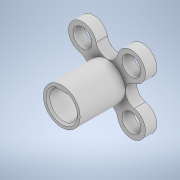
# Autodesk Inventor part: teenee_part
Saved by Autodesk Inventor 2020 (Build 240168000, 168)
## iProperties
Created: 2019-04-24
Part Number: teenee_part
Material: Generic
Document SubType Name: Modeling
Designer: Connor
Density: 1 g/cm^3
Appearance: Default
Author: Connor
Autodesk Inventor part; units mm, degrees
ref_plane "YZ Plane" through (0, 0, 0) normal (1, 0, 0) x (0, 1, 0)
ref_plane "XZ Plane" through (0, 0, 0) normal (0, 1, 0) x (-1, 0, 0)
ref_plane "XY Plane" through (0, 0, 0) normal (0, 0, 1) x (1, 0, 0)
sketch "Sketch1" plane through (0, 0, 0) normal (0, 0, 1) x (1, 0, 0)
  line L0 (-12.5, 12.5) -> (12.5, 12.5)
  line L1 (12.5, 12.5) -> (12.5, -12.5)
  line L2 (12.5, -12.5) -> (-12.5, -12.5)
  line L3 (-12.5, -12.5) -> (-12.5, 12.5)
  line L4 (-12.5, 12.5) -> (12.5, -12.5) construction
  line L5 (-12.5, -12.5) -> (12.5, 12.5) construction
  arc A0 (-1.7861, 2.625) -> (1.7861, 2.625) centre (0, 0) ccw
  line L6 (-1.7861, 2.625) -> (1.7861, 2.625)
  circle A1 centre (-6.5, 6.5) radius 2.5
  circle A2 centre (6.5, 6.5) radius 2.5
  circle A3 centre (6.5, -6.5) radius 2.5
  circle A4 centre (-6.5, -6.5) radius 2.5
  line L7 (1.9339, 3.125) -> (-1.9339, 3.125)
  arc A5 (-1.9339, 3.125) -> (1.9339, 3.125) centre (0, 0) ccw
  point P0 (0, 0)
  dimension "d0" = 6.35
  dimension "d1" = 25
  dimension "d2" = 5.8
  dimension "d3" = 5
  dimension "d6" = 13
  dimension "d7" = 0.5
  constraints: 16 end point, 6 centre point, 4 point on circle, 4 point on line, 3 equal radius, 2 coincident, 2 horizontal, 2 horizontal alignment, 2 parallel, 2 perpendicular, 1 midpoint, 1 vertical alignment, 1 other
  measures "d0" diameter of A0
  measures "d1" distance between parallel lines of L1 L3
  measures "d3" diameter of A1
  measures "d6" distance of A2.centre A1.centre
  measures "d7" radial gap between concentric circles of A0 A5
extrude "Extrusion1" add sketch "Sketch1" along normal blind 3 contours L0 L1 L2 L3
sketch "Sketch2" plane through (0, 0, 3) normal (0, 0, 1) x (1, 0, 0)
  line L0 (12.5, 12.5) -> (-12.5, 12.5) projected
  line L1 (-12.5, 12.5) -> (-12.5, -12.5) projected
  line L2 (-12.5, -12.5) -> (12.5, -12.5) projected
  line L3 (12.5, -12.5) -> (12.5, 12.5) projected
  circle A0 centre (-6.5, 6.5) radius 2.5 projected
  circle A1 centre (6.5, 6.5) radius 2.5 projected
  circle A2 centre (6.5, -6.5) radius 2.5 projected
  circle A3 centre (-6.5, -6.5) radius 2.5 projected
  arc A4 (-1.9339, 3.125) -> (1.9339, 3.125) centre (0, 0) ccw projected
  line L4 (-1.9339, 3.125) -> (1.9339, 3.125) projected
  arc A5 (-2.8723, 7.2281) -> (-7.2281, 2.8723) centre (-6.5, 6.5) ccw
  arc A6 (-7.2281, -2.8723) -> (-2.8723, -7.2281) centre (-6.5, -6.5) ccw
  arc A7 (2.8723, -7.2281) -> (7.2281, -2.8723) centre (6.5, -6.5) ccw
  arc A8 (7.2281, 2.8723) -> (2.8723, 7.2281) centre (6.5, 6.5) ccw
  arc A9 (-7.2281, -2.8723) -> (-7.2281, 2.8723) centre (-7.8046, 0) ccw
  arc A10 (-2.8723, 7.2281) -> (2.8723, 7.2281) centre (0, 7.8046) ccw
  arc A11 (7.2281, 2.8723) -> (7.2281, -2.8723) centre (7.8046, 0) ccw
  arc A12 (2.8723, -7.2281) -> (-2.8723, -7.2281) centre (0, -7.8046) ccw
  point P0 (0, 0)
  dimension "d12" = 1.2
  dimension "d13" = 1.2
  constraints: 16 point on circle, 8 centre point, 8 tangent, 6 equal radius, 4 coincident
  measures "d12" radial gap between concentric circles of A5 A0
extrude "Extrusion2" cut sketch "Sketch2" against normal through all contours L3 L2 L1 L0
sketch "Sketch3" plane through (0, 0, 3) normal (0, 0, 1) x (1, 0, 0)
  arc A0 (-2.8723, 7.2281) -> (-7.2281, 2.8723) centre (-6.5, 6.5) ccw projected
  arc A1 (-7.2281, -2.8723) -> (-7.2281, 2.8723) centre (-7.8046, 0) ccw projected
  arc A2 (-7.2281, -2.8723) -> (-2.8723, -7.2281) centre (-6.5, -6.5) ccw projected
  arc A3 (2.8723, -7.2281) -> (-2.8723, -7.2281) centre (0, -7.8046) ccw projected
  arc A4 (2.8723, -7.2281) -> (7.2281, -2.8723) centre (6.5, -6.5) ccw projected
  arc A5 (7.2281, 2.8723) -> (7.2281, -2.8723) centre (7.8046, 0) ccw projected
  arc A6 (7.2281, 2.8723) -> (2.8723, 7.2281) centre (6.5, 6.5) ccw projected
  arc A7 (-2.8723, 7.2281) -> (2.8723, 7.2281) centre (0, 7.8046) ccw projected
  circle A8 centre (-6.5, 6.5) radius 2.5 projected
  circle A9 centre (6.5, 6.5) radius 2.5 projected
  circle A10 centre (6.5, -6.5) radius 2.5 projected
  circle A11 centre (-6.5, -6.5) radius 2.5 projected
  arc A12 (-1.9339, 3.125) -> (1.9339, 3.125) centre (0, 0) ccw projected
  line L0 (-1.9339, 3.125) -> (1.9339, 3.125) projected
  circle A13 centre (0, 0) radius 4.875
  arc A14 (-7.2281, -2.8723) -> (-7.2281, 2.8723) centre (-7.8046, 0) ccw projected
  point P0 (0, 0)
  constraints: 1 centre point, 1 coincident, 1 tangent
extrude "Extrusion3" add sketch "Sketch3" along normal blind 12 contours A13
chamfer "Chamfer1" distance 0.5 angle 45 2 edges at (0, 3.125, 15) (0, -3.675, 15)
body "Solid1"
